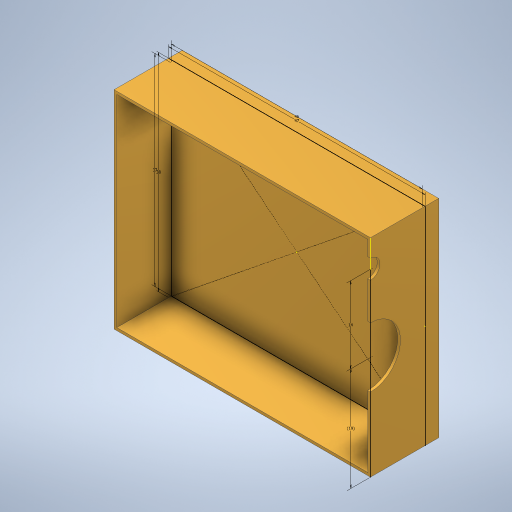
# Autodesk Inventor part: HUDSON-1-54A
Saved by Autodesk Inventor 2024.2 (Build 282272000, 272)
## iProperties
Created: 2024-10-24
Part Number: HUDSON-1-54A
Material: Generic
Document SubType Name: Modeling
Designer: Precisión-05
Density: 1 g/cm^3
Appearance: Default
Author: Precisión-05
Autodesk Inventor part; units mm, degrees
ref_plane "YZ Plane" through (0, 0, 0) normal (1, 0, 0) x (0, 1, 0)
ref_plane "XZ Plane" through (0, 0, 0) normal (0, 1, 0) x (-1, 0, 0)
ref_plane "XY Plane" through (0, 0, 0) normal (0, 0, 1) x (1, 0, 0)
sketch "Sketch1" plane through (0, 0, 0) normal (0, 1, 0) x (-1, 0, 0)
  line L0 (-23.5, -19) -> (23.5, -19)
  line L1 (23.5, -19) -> (23.5, 19)
  line L2 (23.5, 19) -> (-23.5, 19)
  line L3 (-23.5, 19) -> (-23.5, -19)
  line L4 (-23.5, -19) -> (23.5, 19) construction
  line L5 (23.5, -19) -> (-23.5, 19) construction
  line L6 (-23, -18.5) -> (23, -18.5)
  line L7 (23, -18.5) -> (23, 18.5)
  line L8 (23, 18.5) -> (-23, 18.5)
  line L9 (-23, 18.5) -> (-23, -18.5)
  line L10 (-23, -18.5) -> (23, 18.5) construction
  line L11 (23, -18.5) -> (-23, 18.5) construction
  point P0 (0, 0)
  dimension "d0" = 47
  dimension "d1" = 38
  dimension "d2" = 46
  dimension "d3" = 37
  constraints: 24 end point, 4 midpoint, 4 parallel, 2 horizontal, 2 perpendicular
  measures "d0" distance of L2.end L1.end
  measures "d1" distance of L1.end L0.end
  measures "d2" distance of L8.end L7.end
  measures "d3" distance of L7.end L6.end
extrude "Extrusion1" add sketch "Sketch1" along normal blind 2.5 contours L3 L2 L1 L0 | L9 L8 L7 L6
extrude "Extrusion2" add sketch "Sketch1" against normal blind 10
sketch "Sketch2" plane through (23.5, 2.5, 19) normal (1, 0, 0) x (0, 0, -1)
  line L0 (38, -12.5) -> (0, -12.5) projected
  line L1 (38, -12.5) -> (19, -12.5)
  line L2 (19, -12.5) -> (5, -12.5)
  point P0 (19, -2.5)
  dimension "d8" = 19
  dimension "d9" = 14
  constraints: 4 end point, 2 coincident, 1 midpoint, 1 point on line
  measures "d8" distance of L0.start L1.end
  measures "d9" distance of L2.start L2.end
hole "Hole1" at (23.5, -10, 14) direction (-1, 0, 0) diameter 3.5 depth 8
hole "Hole2" at (23.5, -10, 0) direction (-1, 0, 0) diameter 11 depth 8
body "Solid1"
